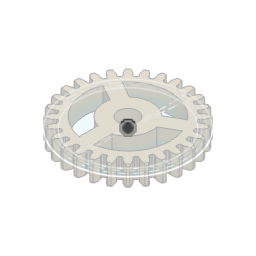
Parametric Spur Gear (Autodesk Fusion 360 design; units mm, degrees)
Autodesk Fusion 360 part; units mm, degrees
sketch "Diameters" plane through (0, 0, 0) normal (0, 1, 0) x (1, 0, 0) in component "Gear"
  circle A0 centre (0, 0) radius 13.1557 construction
  circle A1 centre (0, 0) radius 12.4
  circle A2 centre (0, 0) radius 14 construction
  circle A3 centre (0, 0) radius 15
  line L0 (0, -12.4) -> (0, 15) construction
  line L1 (-1.3884, -12.322) -> (1.6795, 14.9057) construction
  dimension "d1" = 26.3114
  dimension "d44" = 24.8
  dimension "d45" = 28
  dimension "d46" = 30
  dimension "d336" = 6.429
  constraint coincident A0.centre A1.centre
  constraint coincident A1 L0.start
  constraint coincident A3 L0.end
  constraint vertical A0.centre L0.start
  constraint vertical L0
  constraint coincident A1 L1.start
  constraint coincident A3 L1.end
  constraint coincident A0.centre L1
  measures "d1" diameter of A0
  measures "d44" diameter of A1
  measures "d45" diameter of A2
  measures "d46" diameter of A3
  measures "d336" angle of L0 L1
sketch "Gear Half-Tooth" plane through (0, 0, 0) normal (0, 1, 0) x (-1, 0, 0) in component "Gear"
  circle A0 centre (0, 0) radius 12.4
  circle A1 centre (0, 0) radius 13.1557 construction
  circle A2 centre (0, 0) radius 14 construction
  circle A3 centre (0, 0) radius 15
  line L0 (0, 0) -> (1.7403, -13.0401) construction
  line L1 (0, 0) -> (2.8702, -12.8388) construction
  line L2 (0, 0) -> (3.9782, -12.5398) construction
  line L3 (0, 0) -> (5.056, -12.1453) construction
  line L4 (0, 0) -> (6.0953, -11.6585) construction
  line L5 (0, 0) -> (7.0882, -11.0829) construction
  line L6 (0, 0) -> (8.0272, -10.4229) construction
  line L7 (0, 0) -> (8.905, -9.6836) construction
  line L8 (0, 0) -> (9.7151, -8.8707) construction
  line L9 (0, 0) -> (10.4513, -7.9902) construction
  line L10 (1.7403, -13.0401) -> (0.6023, -13.192) construction
  line L11 (2.8702, -12.8388) -> (0.6294, -13.3397) construction
  line L12 (5.056, -12.1453) -> (0.8165, -13.9102) construction
  line L13 (6.0953, -11.6585) -> (1.0083, -14.318) construction
  line L14 (7.0882, -11.0829) -> (1.2852, -14.7942) construction
  line L15 (8.0272, -10.4229) -> (1.6602, -15.3264) construction
  line L16 (8.905, -9.6836) -> (2.1446, -15.9005) construction
  line L17 (9.7151, -8.8707) -> (2.7481, -16.5009) construction
  line L18 (10.4513, -7.9902) -> (3.4786, -17.1106) construction
  line L19 (0, 0) -> (0.5971, -13.1421) construction
  line L20 (3.9782, -12.5398) -> (0.6953, -13.5813) construction
  line L21 (0.5798, -12.7612) -> (0.5971, -13.1421)
  line L22 (0, 0) -> (0.8438, -13.9745) construction
  line L23 (0, 0) -> (0, -15)
  arc A4 (0, -12.4) -> (0.1943, -12.3985) centre (0, 0) ccw
  arc A5 (0.5798, -12.7612) -> (0.1943, -12.3985) centre (0.2002, -12.7784) ccw
  spline S0 degree 5 poles (0.5971, -13.1421) (0.597, -13.1428) (0.5969, -13.1449) (0.5971, -13.1506) (0.5984, -13.163) (0.6014, -13.1864) (0.606, -13.2176) (0.6124, -13.2557) (0.6207, -13.2999) (0.6312, -13.3491) (0.6439, -13.4027) (0.6589, -13.4601) (0.6764, -13.5211) (0.6963, -13.5854) (0.7187, -13.653) (0.7435, -13.7236) (0.7709, -13.797) (0.8008, -13.8729) (0.8333, -13.9511) (0.8684, -14.0313) (0.9061, -14.1134) (0.9465, -14.1972) (0.9895, -14.2826) (1.0351, -14.3695) (1.0834, -14.4578) (1.1343, -14.5474) (1.1879, -14.6381) (1.2441, -14.7299) (1.3029, -14.8226) (1.3644, -14.916) (1.4285, -15.0102) (1.4952, -15.1051) (1.5645, -15.2004) (1.6365, -15.2962) (1.711, -15.3924) (1.788, -15.4889) (1.8677, -15.5856) (1.9499, -15.6825) (2.0346, -15.7794) (2.1219, -15.8764) (2.2117, -15.9734) (2.3039, -16.0703) (2.3987, -16.1669) (2.4959, -16.2633) (2.5955, -16.3594) (2.6975, -16.4551) (2.802, -16.5503) (2.9088, -16.6451) (3.018, -16.7393) (3.1295, -16.833) (3.2433, -16.9261) (3.3363, -17.0002) (3.407, -17.0555) (3.4546, -17.0923) (3.4786, -17.1106) knots 0 0 0 0 0 0 0.02 0.04 0.06 0.08 0.1 0.12 0.14 0.16 0.18 0.2 0.22 0.24 0.26 0.28 0.3 0.32 0.34 0.36 0.38 0.4 0.42 0.44 0.46 0.48 0.5 0.52 0.54 0.56 0.58 0.6 0.62 0.64 0.66 0.68 0.7 0.72 0.74 0.76 0.78 0.8 0.82 0.84 0.86 0.88 0.9 0.92 0.94 0.96 0.98 1 1 1 1 1 1
  point P0 (-2.7481, -16.5009)
  point P1 (-3.4786, -17.1106)
  point P2 (-2.1446, -15.9005)
  point P3 (-1.6602, -15.3264)
  point P4 (-1.2852, -14.7942)
  point P5 (-1.0083, -14.318)
  point P6 (-0.8165, -13.9102)
  point P7 (-0.6953, -13.5813)
  point P8 (-0.6294, -13.3397)
  point P9 (-0.6023, -13.192)
  point P10 (-0.5971, -13.1421)
  dimension "d273" = 5
  dimension "d274" = 5
  dimension "d275" = 5
  dimension "d276" = 5
  dimension "d277" = 5
  dimension "d278" = 5
  dimension "d279" = 5
  dimension "d280" = 5
  dimension "d281" = 5
  dimension "d283" = 1.1481
  dimension "d284" = 2.2961
  dimension "d286" = 4.5922
  dimension "d287" = 5.7403
  dimension "d288" = 6.8883
  dimension "d289" = 8.0364
  dimension "d290" = 9.1844
  dimension "d291" = 10.3325
  dimension "d292" = 11.4805
  dimension "d294" = 5
  dimension "d295" = 3.4442
  dimension "d324" = 3.455
  dimension "d325" = 0.38
  constraint coincident A0.centre A1.centre
  constraint coincident A1 L0.end
  constraint coincident A1 L1.end
  constraint coincident A1 L2.end
  constraint coincident A1 L3.end
  constraint coincident A1 L4.end
  constraint coincident A1 L5.end
  constraint coincident A1 L6.end
  constraint coincident A1 L7.end
  constraint coincident A1 L8.end
  constraint coincident A1 L9.end
  constraint coincident A1 L19.end
  constraint tangent A1 L10
  constraint tangent A1 L11
  constraint tangent A1 L12
  constraint tangent A1 L13
  constraint tangent A1 L14
  constraint tangent A1 L15
  constraint tangent A1 L16
  constraint tangent A1 L17
  constraint tangent A1 L18
  constraint tangent A1 L20
  constraint coincident A2 L22.end
  constraint vertical L23
  constraint coincident L23 A4.start
  constraint tangent A4 A5
  constraint tangent L21 A5
  constraint coincident L19 L21.start
  constraint coincident A0 A4.end
  constraint coincident L22.end S0
  constraint symmetric L17.end L23 P0
  constraint symmetric L10.end L23 P9
  constraint symmetric L11.end L23 P8
  constraint symmetric L12.end L23 P6
  constraint symmetric L13.end L23 P5
  constraint symmetric L14.end L23 P4
  constraint symmetric L15.end L23 P3
  constraint symmetric L16.end L23 P2
  constraint symmetric L18.end L23 P1
  constraint symmetric L19.end L23 P10
  constraint symmetric L20.end L23 P7
  constraint coincident A3 L23.end
  measures "d273" angle of L0 L1
  measures "d274" angle of L1 L2
  measures "d275" angle of L2 L3
  measures "d276" angle of L3 L4
  measures "d277" angle of L4 L5
  measures "d278" angle of L5 L6
  measures "d279" angle of L6 L7
  measures "d280" angle of L7 L8
  measures "d281" angle of L8 L9
  measures "d283" distance of L0.end L10.end
  measures "d284" distance of L1.end L11.end
  measures "d286" distance of L3.end L12.end
  measures "d287" distance of L4.end L13.end
  measures "d288" distance of L5.end L14.end
  measures "d289" distance of L6.end L15.end
  measures "d290" distance of L7.end L16.end
  measures "d291" distance of L8.end L17.end
  measures "d292" distance of L9.end L18.end
  measures "d294" angle of L0 L19
  measures "d295" distance of L2.end L20.end
  measures "d324" angle of L22 L23
  measures "d325" radius of A5
extrude "Create Disc" add sketch "Diameters" along normal mid plane 5 contours A1 | A3 in component "Gear"
chamfer "Chamfer1" distance 0.35 angle 45 2 edges at (-13.9849, 2.5, 5.4242) (-13.9849, -2.5, -5.4242) in component "Gear"
extrude "Create Half-tooth" cut sketch "Gear Half-Tooth" along normal through all and the other way through all contours A0 A3 L21 L23 A4 A5 S0 in component "Gear"
mirror "Create full tooth" about plane through (0, 0, -12.4) normal (-1, 0, 0) of "Create Half-tooth" in component "Gear"
pattern_circular "Replicate half-tooth" count 28 over 360 about axis through (0, -2.5, 0) along (0, 1, 0) of "Create Half-tooth" in component "Gear"
pattern_circular "Replicate full tooth" count 28 over 360 about axis through (0, -2.5, 0) along (0, 1, 0) of "Create full tooth" in component "Gear"
sketch "Hole" plane through (0, -2.5, 0) normal (0, -1, 0) x (-1, 0, 0) in component "Gear"
  circle A0 centre (0, 0) radius 13.75
  circle A1 centre (0, 0) radius 2.5
  circle A2 centre (0, 0) radius 10.6286
  circle A3 centre (0, 0) radius 6.0429
  line L0 (-1.7714, -5.7774) -> (-1.7714, -10.4799)
  line L1 (1.7714, -5.7774) -> (1.7714, -10.4799)
  line L2 (-5.8891, 1.3546) -> (-9.9616, 3.7059)
  line L3 (-4.1176, 4.4228) -> (-8.1902, 6.7741)
  line L4 (5.8891, 1.3546) -> (9.9616, 3.7059)
  line L5 (4.1176, 4.4228) -> (8.1902, 6.7741)
  dimension "d244" = 5
  dimension "d255" = 21.2571
  dimension "d256" = 12.0857
  dimension "d257" = 3.5429
  dimension "d260" = 120
  dimension "d262" = 3.5429
  dimension "d263" = 3.5429
  dimension "d264" = 120
  constraint concentric A0 A1
  constraint concentric A0 A2
  constraint coincident A0.centre A1.centre
  constraint coincident A3 L0.start
  constraint coincident A2 L0.end
  constraint vertical L0
  constraint coincident A3 L1.start
  constraint coincident A2 L1.end
  constraint vertical L1
  constraint equal L0 L1
  constraint coincident A3 L2.start
  constraint coincident A2 L2.end
  constraint coincident A3 L3.start
  constraint coincident A2 L3.end
  constraint equal L2 L3
  constraint coincident A3 L4.start
  constraint coincident A2 L4.end
  constraint coincident A3 L5.start
  constraint coincident A2 L5.end
  constraint equal L4 L5
  constraint parallel L4 L5
  constraint parallel L2 L3
  measures "d244" diameter of A1
  measures "d255" diameter of A2
  measures "d256" diameter of A3
  measures "d257" distance of L0 L1
  measures "d260" angle of L1 L4
  measures "d262" distance of L4 L5
  measures "d263" distance of L2 L3
  measures "d264" angle of L0 L2
extrude "Add Hole" cut sketch "Hole" against normal blind 5 contours A1 in component "Gear"
extrude "Add Slots" cut sketch "Hole" against normal blind 5 contours A2 A3 L1 L4 | A2 A3 L3 L5 | A2 A3 L0 L2 in component "Gear"
component "Gear" placed x (1, 0, 0) y (0, 1, 0) z (0, 0, 1) at (0, 0, 0)
equation "d1 = GEAR_BASE_DIAMETER"
equation "GEAR_BASE_DIAMETER = GEAR_REFERENCE_DIAMETER * cos(GEAR_PRESSURE_ANGLE)"
equation "GEAR_TOOTH_CONSTRUCTION_ANGLE = 5 deg"
equation "GEAR_MODULE = 1"
equation "GEAR_PRESSURE_ANGLE = 20 deg"
equation "GEAR_TEETH = 28"
equation "GEAR_REFERENCE_DIAMETER = ( GEAR_TEETH * GEAR_MODULE ) * 1 mm"
equation "GEAR_TIP_DIAMETER = GEAR_REFERENCE_DIAMETER + ( 2 * GEAR_MODULE ) * 1 mm"
equation "GEAR_ROOT_DIAMETER = GEAR_REFERENCE_DIAMETER - ( 3.2 * GEAR_MODULE ) * 1 mm"
equation "d44 = GEAR_ROOT_DIAMETER"
equation "d45 = GEAR_REFERENCE_DIAMETER"
equation "d46 = GEAR_TIP_DIAMETER"
equation "GEAR_THICKNESS = 5 mm"
equation "GEAR_FILLET_RADIUS = ( 0.38 * GEAR_MODULE ) * 1 mm"
equation "d222 = GEAR_THICKNESS / 2"
equation "GEAR_TOOTH_SCALE = 0.925"
equation "GEAR_HOLE_DIAMETER = 5 mm"
equation "d244 = GEAR_HOLE_DIAMETER"
equation "GEAR_SLOT_WIDTH = GEAR_ROOT_DIAMETER / 7"
equation "d253 = -GEAR_THICKNESS"
equation "d255 = GEAR_ROOT_DIAMETER - GEAR_SLOT_WIDTH"
equation "d256 = GEAR_HOLE_DIAMETER + GEAR_SLOT_WIDTH * 2"
equation "d257 = GEAR_SLOT_WIDTH"
equation "d262 = GEAR_SLOT_WIDTH"
equation "d263 = GEAR_SLOT_WIDTH"
equation "d265 = -GEAR_THICKNESS"
equation "GEAR_TIP_CHAMFER = 0.35 mm"
equation "d273 = GEAR_TOOTH_CONSTRUCTION_ANGLE"
equation "d274 = GEAR_TOOTH_CONSTRUCTION_ANGLE"
equation "d275 = GEAR_TOOTH_CONSTRUCTION_ANGLE"
equation "d276 = GEAR_TOOTH_CONSTRUCTION_ANGLE"
equation "d277 = GEAR_TOOTH_CONSTRUCTION_ANGLE"
equation "d278 = GEAR_TOOTH_CONSTRUCTION_ANGLE"
equation "d279 = GEAR_TOOTH_CONSTRUCTION_ANGLE"
equation "d280 = GEAR_TOOTH_CONSTRUCTION_ANGLE"
equation "d281 = GEAR_TOOTH_CONSTRUCTION_ANGLE"
equation "d283 = ( PI * GEAR_BASE_DIAMETER * GEAR_TOOTH_CONSTRUCTION_ANGLE / 360 deg ) * 1"
equation "d284 = ( PI * GEAR_BASE_DIAMETER * GEAR_TOOTH_CONSTRUCTION_ANGLE / 360 deg ) * 2"
equation "d286 = ( PI * GEAR_BASE_DIAMETER * GEAR_TOOTH_CONSTRUCTION_ANGLE / 360 deg ) * 4"
equation "d287 = ( PI * GEAR_BASE_DIAMETER * GEAR_TOOTH_CONSTRUCTION_ANGLE / 360 deg ) * 5"
equation "d288 = ( PI * GEAR_BASE_DIAMETER * GEAR_TOOTH_CONSTRUCTION_ANGLE / 360 deg ) * 6"
equation "d289 = ( PI * GEAR_BASE_DIAMETER * GEAR_TOOTH_CONSTRUCTION_ANGLE / 360 deg ) * 7"
equation "d290 = ( PI * GEAR_BASE_DIAMETER * GEAR_TOOTH_CONSTRUCTION_ANGLE / 360 deg ) * 8"
equation "d291 = ( PI * GEAR_BASE_DIAMETER * GEAR_TOOTH_CONSTRUCTION_ANGLE / 360 deg ) * 9"
equation "d292 = ( PI * GEAR_BASE_DIAMETER * GEAR_TOOTH_CONSTRUCTION_ANGLE / 360 deg ) * 10"
equation "d294 = GEAR_TOOTH_CONSTRUCTION_ANGLE"
equation "d295 = ( PI * GEAR_BASE_DIAMETER * GEAR_TOOTH_CONSTRUCTION_ANGLE / 360 deg ) * 3"
equation "d324 = ( ( 360 deg / GEAR_TEETH ) * ( 1 - GEAR_TOOTH_SCALE / 2 ) ) / 2"
equation "d325 = GEAR_FILLET_RADIUS"
equation "d327 = GEAR_TEETH"
equation "d333 = GEAR_TEETH"
equation "d335 = GEAR_TIP_CHAMFER"
equation "d336 = 180 deg / GEAR_TEETH"
named bodies: "Gear"
